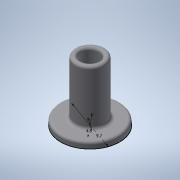
# Autodesk Inventor part: BNC_RG174_AdaptRing_10mm_3mm
Saved by Autodesk Inventor 2022 (Build 260153000, 153)
## iProperties
Created: 2023-03-27
Part Number: BNC_RG174_AdaptRing_10mm_3mm
Material: Generic
Document SubType Name: Modeling
Designer: baaij
Density: 1 g/cm^3
Appearance: Default
Author: baaij
Autodesk Inventor part; units mm, degrees
ref_plane "YZ Plane" through (0, 0, 0) normal (1, 0, 0) x (0, 1, 0)
ref_plane "XZ Plane" through (0, 0, 0) normal (0, 1, 0) x (-1, 0, 0)
ref_plane "XY Plane" through (0, 0, 0) normal (0, 0, 1) x (1, 0, 0)
sketch "Sketch1" plane through (0, 0, 0) normal (0, 0, 1) x (1, 0, 0)
  line L0 (0, 6.79) -> (0, -6.79) construction
  line L1 (-6.79, 0) -> (6.79, 0) construction
  circle A0 centre (0, 0) radius 4.85
  circle A1 centre (0, 0) radius 1.5
  circle A2 centre (0, 0) radius 2.4
  dimension "d4" = 9.7
  dimension "d5" = 3
  dimension "d6" = 4.8
  constraints: 3 centre point, 3 coincident
  measures "d4" diameter of A0
  measures "d5" diameter of A1
  measures "d6" diameter of A2
extrude "Extrusion3" add sketch "Sketch1" along normal blind 1 contours A0
extrude "Extrusion4" add sketch "Sketch1" along normal blind 10 contours A2
fillet "Fillet1" radius 0.3 1 edges at (-1.5, 0, 0)
fillet "Fillet2" radius 0.5 1 edges at (-2.4, 0, 1)
fillet "Fillet3" radius 0.4 1 edges at (-4.85, 0, 1)
fillet "Fillet4" radius 0.4 2 edges at (-2.4, 0, 10) (-1.5, 0, 10)
body "Solid3"
